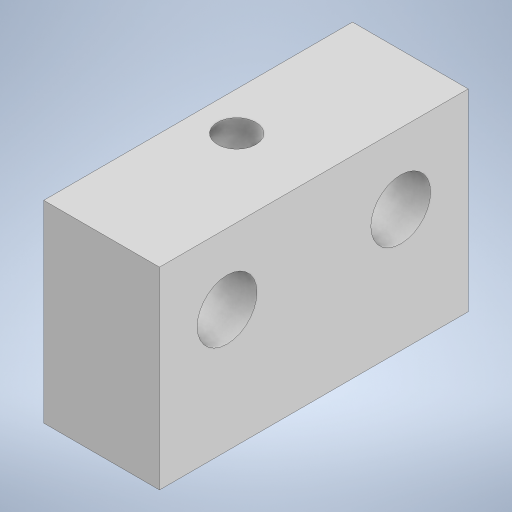
# Autodesk Inventor part: middleFingerMale
Saved by Autodesk Inventor 2024 (Build 280153000, 153)
## iProperties
Created: 2024-06-10
Part Number: middleFingerMale
Material: Generic
Document SubType Name: Modeling
Designer: omiye
Density: 1 g/cm^3
Appearance: Default
Author: omiye
Autodesk Inventor part; units mm, degrees
ref_plane "YZ Plane" through (0, 0, 0) normal (1, 0, 0) x (0, 1, 0)
ref_plane "XZ Plane" through (0, 0, 0) normal (0, 1, 0) x (-1, 0, 0)
ref_plane "XY Plane" through (0, 0, 0) normal (0, 0, 1) x (1, 0, 0)
sketch "Sketch1" plane through (0, 0, 0) normal (0, 1, 0) x (-1, 0, 0)
  line L0 (-3, -8) -> (3, -8)
  line L1 (3, -8) -> (3, 8)
  line L2 (3, 8) -> (-3, 8)
  line L3 (-3, 8) -> (-3, -8)
  line L4 (-3, -8) -> (3, 8) construction
  line L5 (3, -8) -> (-3, 8) construction
  point P0 (0, 0)
  dimension "d0" = 6
  dimension "d1" = 16
  constraints: 12 end point, 2 midpoint, 2 parallel, 1 horizontal, 1 perpendicular
  measures "d0" distance of L2.end L1.end
  measures "d1" distance of L1.end L0.end
extrude "Extrusion1" add sketch "Sketch1" along normal blind 10
sketch "Sketch2" plane through (0, 10, 0) normal (0, 1, 0) x (1, 0, 0)
  line L0 (-3, 8) -> (-3, -8) projected
  line L1 (-3, 0) -> (-1, 0)
  circle A0 centre (-1, 0) radius 1
  point P0 (0, 0)
  dimension "d4" = 2
  dimension "d5" = 2
  constraints: 2 end point, 1 centre point, 1 coincident, 1 horizontal, 1 midpoint
  measures "d4" distance of L1.start L1.end
  measures "d5" diameter of A0
sketch "Sketch3" plane through (3, 0, -8) normal (0, 0, -1) x (-1, 0, 0)
  line L0 (6, 0) -> (6, 10) projected
  line L1 (6, 10) -> (10.4832, 2.2349)
  line L2 (6, 10) -> (14.9664, 10) construction
  point P0 (3, 0)
  dimension "d6" = 60
  constraints: 4 end point, 1 equal length, 1 horizontal
  measures "d6" angle of L1 L2
sweep "Sweep1" cut profiles "Sketch2" path "Sketch3" path curves L1
sketch "Sketch5" plane through (3, 0, 8) normal (1, 0, 0) x (0, 0, -1)
  circle A0 centre (3.5, 6.346) radius 2.85 projected
  circle A1 centre (3.5, 6.346) radius 1.55
  circle A2 centre (12.5, 6.346) radius 2.85 projected
  circle A3 centre (12.5, 6.346) radius 1.55
  point P0 (8, 0)
  dimension "d13" = 3.1
  dimension "d14" = 3.1
  constraints: 2 centre point, 2 coincident
  measures "d13" diameter of A1
  measures "d14" diameter of A3
extrude "Extrusion3" cut sketch "Sketch5" against normal blind 10 contours A1 | A3
body "Solid1"
